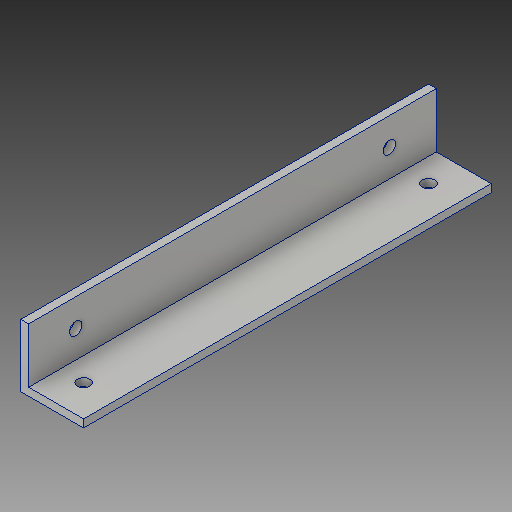
# Autodesk Inventor part: FRA_014_AngleBracketGearbox
Saved by Autodesk Inventor 2018 (Build 220112000, 112)
## iProperties
Created: 2020-01-25
Part Number: FRA_014_AngleBracketGearbox
Material: Aluminum 6061
Document SubType Name: Modeling
Designer: 22barlalex
Density: 2.7 g/cm^3
Appearance: Aluminum - Flat
Mass: 66.7026 g
Surface Area: 171.165 cm^2
Volume: 24.7047 cm^3
Author: 22barlalex
Autodesk Inventor part; units mm, degrees
ref_plane "YZ Plane" through (0, 0, 0) normal (1, 0, 0) x (0, 1, 0)
ref_plane "XZ Plane" through (0, 0, 0) normal (0, 1, 0) x (-1, 0, 0)
ref_plane "XY Plane" through (0, 0, 0) normal (0, 0, 1) x (1, 0, 0)
sketch "Sketch1" plane through (0, 0, 0) normal (0, 0, 1) x (1, 0, 0)
  line L0 (0, 0) -> (3.175, 0)
  line L1 (3.175, 0) -> (3.175, 25.4)
  line L2 (3.175, 25.4) -> (0, 25.4)
  line L3 (0, 25.4) -> (0, 0)
  line L4 (0, 0) -> (25.4, 0)
  line L5 (25.4, 0) -> (25.4, 3.175)
  line L6 (25.4, 3.175) -> (0, 3.175)
  line L7 (0, 3.175) -> (0, 0)
  dimension "d0" = 3.175
  dimension "d1" = 25.4
  constraints: 16 end point, 4 parallel, 4 perpendicular, 2 horizontal
  measures "d0" distance between parallel lines of L1 L3
  measures "d1" distance between parallel lines of L3 L5
extrude "Extrusion1" add sketch "Sketch1" along normal blind 165.1
sketch "Sketch2" plane through (3.175, 3.175, 0) normal (1, 0, 0) x (0, 0, -1)
  line L0 (-165.1, 0) -> (-165.1, 22.225) projected
  line L1 (0, -3.175) -> (-165.1, -3.175) projected
  point P0 (-146.05, 11.1125)
  point P1 (-19.05, 11.1125)
  dimension "d4" = 19.05
  dimension "d5" = 127
  dimension "d6" = 14.2875
  constraints: 1 horizontal alignment
  measures "d4" distance from line of L0 point (-146.05, 11.113)
  measures "d5" distance of point (-19.05, 11.113) point (-146.05, 11.113)
  measures "d6" distance from line of point (-19.05, 11.113) L1
hole "Hole1" at (3.175, 14.2875, 146.05) at (3.175, 14.2875, 19.05) direction (-1, 0, 0) diameter 5.1054 end through all clearance for "Flat Head Machine Screw (82)" size "#10" standard "Ansi Unified Screw Threads"
sketch "Sketch3" plane through (3.175, 3.175, 0) normal (0, 1, 0) x (1, 0, 0)
  line L0 (22.225, 0) -> (0, 0) projected
  line L1 (22.225, 0) -> (22.225, -165.1) projected
  line L2 (0, 0) -> (0, -165.1) projected
  point P0 (-3.175, 0)
  point P1 (9.525, -152.4)
  point P2 (9.525, -12.7)
  dimension "d14" = 12.7
  dimension "d15" = 139.7
  dimension "d16" = 12.7
  dimension "d17" = 9.525
  constraints: 1 vertical alignment
  measures "d14" distance from line of L0 point (9.525, -12.7)
  measures "d15" distance of point (9.525, -152.4) point (9.525, -12.7)
  measures "d16" distance from line of L1 point (9.525, -152.4)
  measures "d17" distance from line of L2 point (9.525, -152.4)
hole "Hole2" at (12.7, 3.175, 152.4) at (12.7, 3.175, 12.7) direction (0, -1, 0) diameter 5.1054 end through all clearance for "Flat Head Machine Screw (82)" size "#10" standard "Ansi Unified Screw Threads"
body "Solid1"
